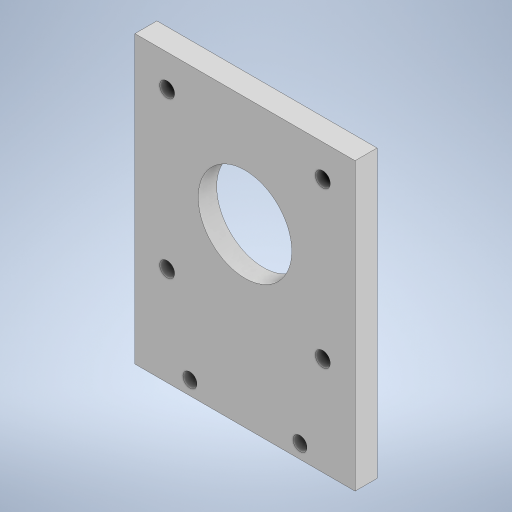
# Autodesk Inventor part: FloorMount
Saved by Autodesk Inventor 2024 (Build 280153000, 153)
## iProperties
Created: 2024-02-13
Part Number: FloorMount
Material: Generic
Document SubType Name: Modeling
Designer: yusuf
Density: 1 g/cm^3
Appearance: Default
Author: yusuf
Autodesk Inventor part; units mm, degrees
ref_plane "YZ Plane" through (0, 0, 0) normal (1, 0, 0) x (0, 1, 0)
ref_plane "XZ Plane" through (0, 0, 0) normal (0, 1, 0) x (-1, 0, 0)
ref_plane "XY Plane" through (0, 0, 0) normal (0, 0, 1) x (1, 0, 0)
sketch "Sketch1" plane through (0, 0, 0) normal (0, 0, 1) x (1, 0, 0)
  line L0 (0, 0) -> (200, 0)
  line L1 (200, 0) -> (200, 260)
  line L2 (200, 260) -> (0, 260)
  line L3 (0, 260) -> (0, 0)
  dimension "d0" = 200
  dimension "d1" = 260
  constraints: 8 end point, 2 parallel, 1 horizontal, 1 perpendicular
  measures "d0" distance of L1.end L2.end
  measures "d1" distance of L0.end L1.end
extrude "Extrusion1" add sketch "Sketch1" along normal blind 20
sketch "Sketch2" plane through (0, 0, 20) normal (0, 0, 1) x (1, 0, 0)
  circle A0 centre (100, 160) radius 42.5
  line L0 (200, 260) -> (0, 260) projected
  line L1 (0, 260) -> (0, 0) projected
  dimension "d4" = 85
  dimension "d5" = 100
  dimension "d6" = 100
  constraints: 1 centre point
  measures "d4" diameter of A0
  measures "d5" distance from line of A0.centre L0
  measures "d6" distance from line of L1 A0.centre
extrude "Extrusion2" cut sketch "Sketch2" against normal blind 30
sketch "Sketch6" plane through (0, 0, 0) normal (0, 0, -1) x (-1, 0, 0)
  circle A0 centre (-29.289, 230.711) radius 6.75
  circle A1 centre (-170.711, 230.711) radius 6.75
  circle A2 centre (-170.711, 89.289) radius 6.75
  circle A3 centre (-29.289, 89.289) radius 6.75
  circle A4 centre (-100, 160) radius 42.5 projected
  circle A5 centre (-50.0126, 12.4968) radius 6.35
  circle A6 centre (-149.9874, 12.4968) radius 6.35
  line L0 (-200, 0) -> (-200, 260) projected
  line L1 (0, 260) -> (0, 0) projected
  line L2 (0, 0) -> (-200, 0) projected
  dimension "d18" = 70.711
  dimension "d19" = 70.711
  dimension "d20" = 70.711
  dimension "d21" = 70.711
  dimension "d22" = 70.711
  dimension "d23" = 70.711
  dimension "d24" = 70.711
  dimension "d25" = 70.711
  dimension "d26" = 13.5
  dimension "d27" = 13.5
  dimension "d28" = 13.5
  dimension "d29" = 13.5
  dimension "d57" = 12.7
  dimension "d58" = 12.7
  dimension "d59" = 50.0126
  dimension "d60" = 50.0126
  dimension "d61" = 12.4968
  dimension "d62" = 12.4968
  constraints: 6 centre point
  measures "d18" horizontal distance of A4.centre A2.centre
  measures "d19" horizontal distance of A4.centre A2.centre
  measures "d20" horizontal distance of A4.centre A1.centre
  measures "d21" horizontal distance of A4.centre A1.centre
  measures "d22" horizontal distance of A4.centre A0.centre
  measures "d23" horizontal distance of A4.centre A0.centre
  measures "d24" horizontal distance of A4.centre A3.centre
  measures "d25" horizontal distance of A4.centre A3.centre
  measures "d26" diameter of A1
  measures "d27" diameter of A0
  measures "d28" diameter of A3
  measures "d29" diameter of A2
  measures "d57" diameter of A6
  measures "d58" diameter of A5
  measures "d59" distance from line of L0 A6.centre
  measures "d60" distance from line of L1 A5.centre
  measures "d61" distance from line of L2 A6.centre
  measures "d62" distance from line of L2 A5.centre
extrude "Extrusion6" cut sketch "Sketch6" against normal blind 20 contours A0 | A1 | A2 | A3 | A5 | A6
sketch "Sketch11" plane through (0, 0, 0) normal (0, 0, -1) x (-1, 0, 0)
  circle A0 centre (-100, 160) radius 42.5 projected
  circle A1 centre (-100, 160) radius 57.15
  point P0 (0, 0)
  dimension "d63" = 114.3
  constraints: 1 centre point, 1 coincident
  measures "d63" diameter of A1
extrude "Extrusion10" cut sketch "Sketch11" against normal blind 3.2
equation "\"d19\" = d18"
equation "\"d20\" = d18"
equation "\"d21\" = d19"
equation "\"d22\" = d20"
equation "\"d23\" = d22"
equation "\"d24\" = d23"
equation "\"d25\" = d23"
equation "\"d58\" = d57"
body "Solid1"
